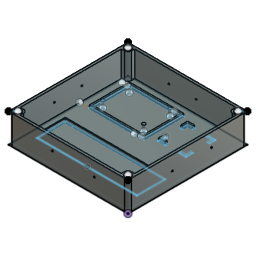
thermal v7 (Autodesk Fusion 360 design; units mm, degrees)
Autodesk Fusion 360 part; units mm, degrees
sketch "Sketch1" plane through (0, 0, 0) normal (0, 1, 0) x (1, 0, 0)
  line L0 (0, 0) -> (-70, 0)
  line L1 (-70, 0) -> (-70, 70)
  line L2 (-70, 70) -> (0, 70)
  line L3 (0, 70) -> (0, 0)
  dimension "d1" = 70
  dimension "d2" = 70
  constraint horizontal L0
  constraint vertical L1
  constraint horizontal L2
  constraint vertical L3
  constraint coincident L0.start L3.end
  measures "d1" distance of L0.start L0.end
  measures "d2" distance of L0.start L2.end
extrude "Extrude1" add sketch "Sketch1" along normal blind 2
sketch "Sketch2" plane through (0, 2, 0) normal (0, 1, 0) x (-1, 0, 0)
  line L0 (0, -70) -> (70, -70)
  line L1 (70, -70) -> (70, 0)
  line L2 (70, 0) -> (0, 0)
  line L3 (0, 0) -> (0, -70)
  line L4 (62.0012, -62.7393) -> (32.0012, -62.7393)
  line L5 (32.0012, -62.7393) -> (32.0012, -41.2393)
  line L6 (32.0012, -41.2393) -> (62.0012, -41.2393)
  line L7 (62.0012, -41.2393) -> (62.0012, -62.7393)
  line L8 (13.8147, -60) -> (11, -60)
  line L9 (25, -45) -> (25, -47.8147)
  line L10 (62.0012, -62.7393) -> (63.4154, -62.7393) construction
  line L11 (32.0012, -41.2393) -> (33.4154, -41.2393) construction
  line L12 (63.0012, -63.7393) -> (31.0012, -63.7393)
  line L13 (31.0012, -63.7393) -> (31.0012, -40.2393)
  line L14 (31.0012, -40.2393) -> (63.0012, -40.2393)
  line L15 (63.0012, -40.2393) -> (63.0012, -63.7393)
  line L16 (13.8147, -61) -> (9.8147, -61)
  line L17 (26, -43.8147) -> (26, -47.8147)
  line L18 (62.0012, -62.7393) -> (66.2472, -62.7393) construction
  circle A0 centre (58.9988, -59.7369) radius 1
  line L19 (26, -61) -> (22, -61)
  line L20 (9.8147, -61) -> (13.8147, -61)
  line L21 (13.8147, -61) -> (13.8147, -60)
  line L22 (9.8147, -61) -> (9.8147, -57.5477)
  line L23 (9.8147, -57.5477) -> (11, -57.5477)
  line L24 (9.8147, -43.8147) -> (9.8147, -47.8147)
  line L25 (11, -47.8147) -> (9.8147, -47.8147)
  line L26 (9.8147, -43.8147) -> (13.8147, -43.8147)
  line L27 (13.8147, -45) -> (13.8147, -43.8147)
  line L28 (26, -43.8147) -> (22, -43.8147)
  line L29 (22, -43.8147) -> (22, -45)
  line L30 (26, -43.8147) -> (26, -47.8147)
  line L31 (25, -47.8147) -> (26.1763, -47.8147)
  line L32 (11, -45) -> (13.8147, -45)
  line L33 (22, -45) -> (25, -45)
  line L34 (9.8147, -43.8147) -> (13.8147, -43.8147)
  line L35 (22, -43.8147) -> (26, -43.8147)
  line L36 (26, -61) -> (26, -57)
  line L37 (26, -57) -> (25, -57)
  line L38 (25, -57) -> (25, -60)
  line L39 (22, -61) -> (22, -60)
  line L40 (22, -60) -> (25, -60)
  line L41 (9.8147, -61) -> (9.8147, -57.5477)
  line L42 (9.8147, -47.8147) -> (9.8147, -43.8147)
  line L43 (11, -60) -> (11, -57.5477)
  line L44 (11, -47.8147) -> (11, -45)
  line L45 (33.8182, -10.0332) -> (4.8182, -10.0332)
  line L46 (58.5866, -26.0332) -> (4.8182, -26.0332)
  line L47 (33.8182, -9.5332) -> (4.3182, -9.5332)
  line L48 (4.8182, -10.0332) -> (62.8182, -10.0332)
  line L49 (63.3182, -26.5332) -> (4.3182, -26.5332)
  line L50 (4.8182, -16.9457) -> (4.8182, -10.0332)
  line L51 (4.3182, -26.5332) -> (4.3182, -9.5332)
  line L52 (58.5866, -26.0332) -> (62.8182, -26.0332)
  line L53 (63.3182, -9.5332) -> (63.3182, -26.5332)
  line L54 (4.8182, -16.9457) -> (4.8182, -26.0332)
  line L55 (33.8182, -9.5332) -> (63.3182, -9.5332)
  line L56 (62.8182, -19.4958) -> (62.8182, -10.0332)
  line L57 (33.8182, -10.0332) -> (62.8182, -10.0332)
  line L58 (62.8182, -19.4958) -> (62.8182, -26.0332)
  line L59 (33.8182, -10.0332) -> (33.8182, -9.5332)
  line L60 (31.0012, -40.2393) -> (36.6612, -40.2393) construction
  circle A1 centre (35.0034, -44.2415) radius 1
  line L61 (63.0012, -40.2393) -> (68.6612, -40.2393) construction
  line L62 (31.0012, -63.7393) -> (36.6612, -63.7393) construction
  circle A2 centre (35.0034, -59.7371) radius 1
  circle A3 centre (58.9989, -44.2415) radius 1
  point P0 (33.8182, -10.0332)
  dimension "d5" = 30
  dimension "d6" = 21.5
  dimension "d7" = 14
  dimension "d8" = 15
  dimension "d9" = 1.4142
  dimension "d12" = 1.4142
  dimension "d14" = 4.246
  dimension "d15" = 2
  dimension "d34" = 4
  dimension "d35" = 4
  dimension "d36" = 4
  dimension "d37" = 4
  dimension "d38" = 4
  dimension "d39" = 4
  dimension "d72" = 0.5
  dimension "d76" = 5.66
  dimension "d77" = 2
  dimension "d79" = 5.66
  dimension "d80" = 5.66
  dimension "d82" = 2
  dimension "d83" = 2
  constraint horizontal L4
  constraint vertical L5
  constraint horizontal L6
  constraint vertical L7
  constraint horizontal L8
  constraint vertical L43
  constraint horizontal L32
  constraint vertical L9
  constraint horizontal L10
  constraint horizontal L11
  constraint horizontal L12
  constraint vertical L13
  constraint horizontal L14
  constraint vertical L15
  constraint horizontal L16
  constraint vertical L41
  constraint horizontal L34
  constraint vertical L17
  constraint horizontal L18
  constraint coincident L16 L19.end
  constraint perpendicular L20 L41
  constraint perpendicular L20 L21
  constraint perpendicular L23 L43
  constraint coincident L24.end L41
  constraint coincident L25.start L43
  constraint perpendicular L24 L25
  constraint perpendicular L27 L34
  constraint coincident L28.end L34
  constraint coincident L29.end L32
  constraint perpendicular L29 L32
  constraint perpendicular L30 L31
  constraint collinear L32 L33
  constraint collinear L34 L35
  constraint perpendicular L19 L36
  constraint perpendicular L36 L37
  constraint perpendicular L8 L38
  constraint perpendicular L19 L39
  constraint collinear L41 L42
  constraint collinear L43 L44
  constraint horizontal L49
  constraint perpendicular L49 L51
  constraint parallel L51 L53
  constraint perpendicular L52 L53
  constraint perpendicular L49 L58
  constraint perpendicular L46 L51
  constraint perpendicular L49 L54
  constraint perpendicular L48 L56
  constraint coincident P0 L45.start
  constraint perpendicular L45 L51
  constraint perpendicular L53 L55
  constraint perpendicular L47 L51
  constraint horizontal L60
  constraint horizontal L61
  constraint horizontal L62
  measures "d5" distance of L4.start L4.end
  measures "d6" distance of L4.start L6.end
  measures "d7" distance of L38.end L8.end
  measures "d8" distance of L38.end L9.start
  measures "d9" distance of L4.start L12.start
  measures "d12" distance of L5.end L13.end
  measures "d14" distance of L4.start A0.centre
  measures "d15" diameter of A0
  measures "d34" distance of L16.end L16.start
  measures "d35" distance of L24.start L24.end
  measures "d36" distance of L24.start L26.end
  measures "d37" distance of L17.start L28.end
  measures "d38" distance of L17.start L17.end
  measures "d39" distance of L19.start L36.end
  measures "d72" distance of L47.start P0
  measures "d76" distance of L13.end A1.centre
  measures "d77" diameter of A1
  measures "d79" distance of L14.end A3.centre
  measures "d80" distance of L12.end A2.centre
  measures "d82" diameter of A2
  measures "d83" diameter of A3
extrude "Extrude2" add sketch "Sketch2" along normal blind 4 contours A0
extrude "Extrude7" add sketch "Sketch2" along normal blind 4 contours A1 | A2 | A3
extrude "Extrude3" add sketch "Sketch2" along normal blind 1.5 contours L12 L13 L14 L15
extrude "Extrude4" add sketch "Sketch2" along normal blind 1.5 contours L8 L16 L20 L21 L22 L23 L41 L43 | L9 L17 L28 L29 L30 L31 L33 L35 | L19 L36 L37 L38 L39 L40 | L24 L25 L26 L27 L32 L34 L42 L44
sketch "Sketch3" plane through (0, 2, 0) normal (0, 1, 0) x (-1, 0, 0)
  line L0 (70, -70) -> (74, -70) construction
  line L1 (0, 0) -> (4, 0) construction
  line L2 (64.5858, -68.5858) -> (5.4142, -68.5858)
  line L3 (1.4142, -64.5858) -> (1.4142, -5.4142)
  line L4 (5.4142, -1.4142) -> (64.5858, -1.4142)
  line L5 (68.5858, -5.4142) -> (68.5858, -64.5858)
  line L6 (5.4142, -1.4142) -> (5.4142, -5.4142)
  line L7 (1.4142, -5.5403) -> (1.4142, -5.4142)
  line L8 (5.4142, -1.4142) -> (5.4142, -5.4142)
  line L9 (5.4142, -5.4142) -> (1.4142, -5.4142)
  line L10 (64.5858, -1.4142) -> (64.5858, -5.4142)
  line L11 (64.5858, -5.4142) -> (68.5858, -5.4142)
  line L12 (64.5858, -68.5858) -> (64.5858, -64.5858)
  line L13 (64.5858, -64.5858) -> (68.5858, -64.5858)
  line L14 (5.4142, -68.5858) -> (5.4142, -64.5858)
  line L15 (5.4142, -64.5858) -> (1.4142, -64.5858)
  line L16 (0, 0) -> (70, 0)
  line L17 (70, 0) -> (70, -70)
  line L18 (70, -70) -> (0, -70)
  line L19 (0, -70) -> (0, 0)
  constraint horizontal L0
  constraint horizontal L1
  constraint coincident L1.start L16.start
  constraint horizontal L2
  constraint vertical L3
  constraint horizontal L4
  constraint vertical L5
  constraint vertical L6
  constraint vertical L7
  constraint vertical L8
  constraint horizontal L9
  constraint vertical L10
  constraint horizontal L11
  constraint vertical L12
  constraint horizontal L13
  constraint vertical L14
  constraint horizontal L15
  constraint horizontal L16
  constraint vertical L17
  constraint horizontal L18
  constraint vertical L19
extrude "Extrude5" add sketch "Sketch3" along normal blind 15
hole "Hole1" at (-1.4142, 9.0391, -48.9799) direction (1, 0, 0) diameter 1 depth 14 tip angle 180
hole "Hole2" at (-1.4142, 8.6563, -26.0128) direction (1, 0, 0) diameter 1 depth 14 tip angle 180
hole "Hole3" at (-19.7207, 8.7497, -1.4142) direction (0, 0, 1) diameter 1 depth 14 tip angle 180
hole "Hole4" at (-44.3914, 9.679, -1.4142) direction (0, 0, 1) diameter 1 depth 14 tip angle 180
hole "Hole5" at (-68.5858, 9.867, -41.5184) direction (-1, 0, 0) diameter 1 depth 14 tip angle 180
hole "Hole6" at (-68.5858, 9.5121, -25.466) direction (-1, 0, 0) diameter 1 depth 14 tip angle 180
hole "Hole7" at (-44.6422, 9.2674, -68.5858) direction (0, 0, -1) diameter 1 depth 14 tip angle 180
hole "Hole8" at (-28.6065, 9.472, -68.5858) direction (0, 0, -1) diameter 1 depth 14 tip angle 180
sketch "Sketch4" plane through (0, 17, 0) normal (0, 1, 0) x (-1, 0, 0)
  line L0 (64.5858, -64.5858) -> (64.5858, -68.5858)
  line L1 (64.5858, -68.5858) -> (5.4142, -68.5858)
  line L2 (5.4142, -68.5858) -> (5.4142, -64.5858)
  line L3 (5.4142, -64.5858) -> (1.4142, -64.5858)
  line L4 (1.4142, -64.5858) -> (1.4142, -5.4142)
  line L5 (1.4142, -5.4142) -> (5.4142, -5.4142)
  line L6 (5.4142, -5.4142) -> (5.4142, -1.4142)
  line L7 (5.4142, -1.4142) -> (64.5858, -1.4142)
  line L8 (64.5858, -1.4142) -> (64.5858, -5.4142)
  line L9 (64.5858, -5.4142) -> (68.5858, -5.4142)
  line L10 (68.5858, -5.4142) -> (68.5858, -64.5858)
  line L11 (68.5858, -64.5858) -> (64.5858, -64.5858)
  line L12 (0, -70) -> (70, -70)
  line L13 (70, -70) -> (70, 0)
  line L14 (70, 0) -> (0, 0)
  line L15 (0, 0) -> (0, -70)
  line L16 (70, 0) -> (67.2928, -2.7072)
  line L17 (0, 0) -> (2.7072, -2.7072)
  line L18 (0, -70) -> (2.7071, -67.2929)
  line L19 (70, -70) -> (67.2929, -67.2929)
  dimension "d67" = 3.8285
  dimension "d68" = 3.8285
  constraint coincident L13.end L14.start
  constraint coincident L12.end L13.start
  constraint coincident L12.start L15.end
  constraint coincident L14.end L15.start
  measures "d67" distance of L13.end L16.end
  measures "d68" distance of L14.end L17.end
hole "Hole9" at (-2.7072, 17, -2.7072) at (-67.2928, 17, -2.7072) at (-67.2929, 17, -67.2929) at (-2.7071, 17, -67.2929) direction (0, -1, 0) diameter 4 depth 14 tip angle 180
sketch "Sketch5" plane through (0, 2, 0) normal (0, 1, 0) x (-1, 0, 0)
extrude "Extrude6" add sketch "Sketch2" along normal blind 2 contours L47 L49 L51 L53 L55
fillet "Fillet1" radius 2 1 edges at (-64.5858, 9.5, -64.5858)
fillet "Fillet2" radius 2 3 edges at (-5.4142, 9.5, -5.4142) (-5.4142, 9.5, -64.5858) (-64.5858, 9.5, -5.4142)
fillet "Fillet3" radius 2 3 edges at (-70, 8.5, -70) (0, 8.5, -70) (-70, 8.5, 0)
fillet "Fillet4" radius 2 1 edges at (0, 8.5, 0)
equation "d9 = ( sqrt(2) ) * 1 mm"
equation "d12 = ( sqrt(2) ) * 1 mm"
equation "d67 = 7.657 mm / 2"
equation "d68 = 7.657 mm / 2"
